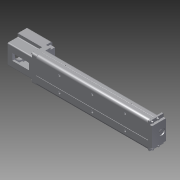
# Autodesk Inventor part: KR45HA-340L-0A0-Body
Saved by Autodesk Inventor 2011 SP1 (Build 150282100, 282)
## iProperties
Created: 2013-10-24
Part Number: KR45HA-340L-0A0-Body
Catalog Web Link: www.cadenas.de
Description: LM Guide Actuator - Body-KR
Vendor: THK
Document SubType Name: Modeling
Designer: PARTuser1
Manufacturer: THK
Density: 1 g/cm^3
Category: PARTsolutions
Company: THK
Title: KR45HA-340L-0A0-Body
Author: Cadenas PARTsolutions
Comments: KR
PSOL_IDENT_0: {$CADENAS_DATA\23d-libs\thk\lm_guide_actuator\type_kr\parts\lm_g_a_kr_body.prj},216 {VTYP=3D},{NB=KR
PSOL_IDENT_1: 45HA-340L-0A0-Body},{LINA=KR45HA-340L-0A0-Body},{NN=LM Guide Actuator - Body},{DATE=10.01.2013 04:45
PSOL_IDENT_2: :24},{GEOMDATE=10.01.2013 04:45:00},{VERSION=},{LINEID=60},{LINESUBID=-1},{WBVAR=LM,TYPE,PC,TOHIF}
PSOL_IDENT_3: {NB=KR45HA-340L-0A0-Body},{LINA=KR45HA-340L-0A0-Body},{KT=DUMMY},{ORDER=KR45H},{XTYPE=6},{LM=340},{L
PSOL_IDENT_4: 1=440},{TYPE=A},{SR=213},{H=70},{G=0},{F=200},{N=3},{N1=2},{LM1=340,440,540,640,740,840,940},{TYPE1=
PSOL_IDENT_5: 'A','B','C','D'},{TYPE2=1},{PC=0},{TOHIF=A0},{TOHIF1='A0','Basic Type (with Housing A, without Inter
PSOL_IDENT_6: mediate flange)','00','Old Basic Type (with Housing A, without Intermediate flange)','0A','Administr
PSOL_IDENT_7: ation number 0A','0B','Administration number 0B','0C','Administration number 0C','0D','Administratio
PSOL_IDENT_8: n number 0D','0F','Administration number 0F'},{TOB=1},{DMTR=64},{A=90},{L=336}
CNS_NT: KR
CNS_NB: KR45HA-340L-0A0-Body
CNS_NBSYN: $ORDER.$TYPE.-$LM.L-$PC.$TOHIF.-Body
CNS_LINA: KR45HA-340L-0A0-Body
CNS_ORDER: KR45H
CNS_XTYPE: 6
CNS_LM: 340
CNS_L1: 440.000
CNS_TYPE: A
CNS_SR: 213.000
CNS_H: 70.000
CNS_G: 0.000
CNS_F: 200.000
CNS_N: 3.000
CNS_N1: 2.000
CNS_LM1: 340,440,540,640,740,840,940
CNS_TYPE1: 'A','B','C','D'
CNS_TYPE2: 1.000
CNS_TOHIF: Basic Type (with Housing A, without Intermediate flange)
CNS_TOHIF1: 'A0','Basic Type (with Housing A, without Intermediate flange)','00','Old Basic Type (with Housing A, without Intermediate flange)','0A','Administration number 0A','0B','Administration number 0B','0C','Administration number 0C','0D','Administration number 0D','0F','Administration number 0F'
CNS_TOB: 1.000
CNS_DMTR: 64.000
CNS_A: 90.000
CNS_L: 336.000
SUPPLIER: THK
ARTICLENO: KR45HA-340L-0A0-Body
BOMINFO: KR45HA-340L-0A0-Body
CREATOR: CADENAS GmbH
Autodesk Inventor part; units mm, degrees
sketch "Sketch_1" plane through (0, 0, 0) normal (1, 0, 0) x (0, 1, 0)
  arc A0 (-22.54, 40) -> (-30.5, 32.04) centre (-22.54, 32.04) ccw
  line L0 (-30.5, 32.04) -> (-30.5, 13)
  line L1 (-30.5, 13) -> (-30, 12.5)
  line L2 (-30, 12.5) -> (-30, -12.5)
  line L3 (-30, -12.5) -> (-30.5, -13)
  line L4 (-30.5, -13) -> (-30.5, -32.04)
  arc A1 (-30.5, -32.04) -> (-22.54, -40) centre (-22.54, -32.04) ccw
  line L5 (-22.54, -40) -> (-15.7, -40)
  line L6 (-15.7, -40) -> (-15.5, -39.8)
  line L7 (-15.5, -39.8) -> (-14.3718, -39.8)
  arc A2 (-12.6282, -39.8) -> (-14.3718, -39.8) centre (-13.5, -41.6) ccw
  line L8 (-12.6282, -39.8) -> (-4.5, -39.8)
  arc A3 (-4.5, -39.8) -> (1.5, -33.8) centre (-4.5, -33.8) ccw
  line L9 (1.5, -33.8) -> (1.5, -29.82)
  line L10 (1.5, -29.82) -> (0.7, -29.02)
  line L11 (0.7, -29.02) -> (-0.6, -29.02)
  line L12 (-0.6, -29.02) -> (-2.75, -31.17)
  line L13 (-2.75, -31.17) -> (-14.25, -31.17)
  line L14 (-14.25, -31.17) -> (-16.4, -29.02)
  line L15 (-16.4, -29.02) -> (-16.5, -29.02)
  arc A4 (-20.5, -25.02) -> (-16.5, -29.02) centre (-16.5, -25.02) ccw
  line L16 (-20.5, -25.02) -> (-20.5, 25.02)
  arc A5 (-16.5, 29.02) -> (-20.5, 25.02) centre (-16.5, 25.02) ccw
  line L17 (-16.5, 29.02) -> (-16.4, 29.02)
  line L18 (-16.4, 29.02) -> (-14.25, 31.17)
  line L19 (-14.25, 31.17) -> (-2.75, 31.17)
  line L20 (-2.75, 31.17) -> (-0.6, 29.02)
  line L21 (-0.6, 29.02) -> (0.7, 29.02)
  line L22 (0.7, 29.02) -> (1.5, 29.82)
  line L23 (1.5, 29.82) -> (1.5, 33.8)
  arc A6 (1.5, 33.8) -> (-4.5, 39.8) centre (-4.5, 33.8) ccw
  line L24 (-4.5, 39.8) -> (-12.6282, 39.8)
  arc A7 (-14.3718, 39.8) -> (-12.6282, 39.8) centre (-13.5, 41.6) ccw
  line L25 (-14.3718, 39.8) -> (-15.5, 39.8)
  line L26 (-15.5, 39.8) -> (-15.7, 40)
  line L27 (-15.7, 40) -> (-22.54, 40)
  constraints: 56 end point, 16 point on circle, 8 centre point
extrude "Extrusion1" add sketch "Sketch_1" along normal blind 340
sketch "Sketch_2" plane through (0, 0, 0) normal (1, 0, 0) x (0, 1, 0)
  line L0 (13, 39.8) -> (-25, 39.8)
  arc A0 (-25, 39.8) -> (-30, 34.8) centre (-25, 34.8) ccw
  line L1 (-30, 34.8) -> (-30, -34.8)
  arc A1 (-30, -34.8) -> (-25, -39.8) centre (-25, -34.8) ccw
  line L2 (-25, -39.8) -> (13, -39.8)
  line L3 (13, -39.8) -> (13, -34)
  line L4 (13, -34) -> (25.75, -34)
  arc A2 (25.75, -34) -> (26.75, -33) centre (25.75, -33) ccw
  line L5 (26.75, -33) -> (26.75, 33)
  arc A3 (26.75, 33) -> (25.75, 34) centre (25.75, 33) ccw
  line L6 (25.75, 34) -> (13, 34)
  line L7 (13, 34) -> (13, 39.8)
  constraints: 16 end point, 8 point on circle, 4 centre point
extrude "Extrusion2" add sketch "Sketch_2" against normal blind 14
sketch "Sketch_3" plane through (0, 0, 0) normal (1, 0, 0) x (0, 1, 0)
  arc A0 (16, 16.52) -> (-16, 16.52) centre (0, -0.0027) ccw
  line L0 (-16, 16.52) -> (-16, -16.52)
  arc A1 (-16, -16.52) -> (16, -16.52) centre (0, 0.0027) ccw
  line L1 (16, -16.52) -> (16, 16.52)
  constraints: 4 end point, 4 point on circle, 2 centre point
extrude "Extrusion3" add sketch "Sketch_3" along normal blind 3.4
sketch "Sketch_4" plane through (0, 0, 0) normal (1, 0, 0) x (0, 1, 0)
  arc A0 (4.5, 22.0454) -> (-16, 15.8193) centre (0, 0) ccw
  line L0 (-16, 15.8193) -> (-16, -15.8193)
  arc A1 (-16, -15.8193) -> (4.5, -22.0454) centre (0, 0) ccw
  line L1 (4.5, -22.0454) -> (4.5, -9.4868)
  arc A2 (4.5, 9.4868) -> (4.5, -9.4868) centre (0, 0) ccw
  line L2 (4.5, 9.4868) -> (4.5, 22.0454)
  constraints: 6 end point, 6 point on circle, 3 centre point
extrude "Extrusion4" add sketch "Sketch_4" along normal blind 12.4
sketch "Sketch_38" plane through (0, 9, 0) normal (0, 1, 0) x (1, 0, 0)
  line L0 (7.4, -15.6) -> (3.4, -15.6)
  line L1 (3.4, -15.6) -> (3.4, -12.1)
  line L2 (3.4, -12.1) -> (7.2, -12.1)
  arc A0 (7.4, -12.3) -> (7.2, -12.1) centre (7.2, -12.3) ccw
  line L3 (7.4, -12.3) -> (7.4, -15.6)
  line L4 (7.4, -15.6) -> (3.4, -15.6)
  constraints: 10 end point, 2 point on circle, 1 centre point
revolve "Revolution1" add sketch "Sketch_38" angle 360 about axis through (7.4, 9, 15.6) along (1, 0, 0)
sketch "Sketch_5" plane through (0, 9, 0) normal (0, 1, 0) x (1, 0, 0)
  line L0 (7.4, 15.6) -> (3.4, 15.6)
  line L1 (3.4, 15.6) -> (3.4, 19.1)
  line L2 (3.4, 19.1) -> (7.2, 19.1)
  arc A0 (7.4, 18.9) -> (7.2, 19.1) centre (7.2, 18.9) ccw
  line L3 (7.4, 18.9) -> (7.4, 15.6)
  line L4 (7.4, 15.6) -> (3.4, 15.6)
  constraints: 10 end point, 2 point on circle, 1 centre point
revolve "Revolution2" add sketch "Sketch_5" angle 360 about axis through (7.4, 9, -15.6) along (1, 0, 0)
sketch "Sketch_7" plane through (340, 0, 0) normal (1, 0, 0) x (0, 0, -1)
  line L0 (-39.8, 11.25) -> (-39.8, -29.25)
  arc A0 (-39.8, -29.25) -> (-39.05, -30) centre (-39.05, -29.25) ccw
  line L1 (-39.05, -30) -> (39.05, -30)
  arc A1 (39.05, -30) -> (39.8, -29.25) centre (39.05, -29.25) ccw
  line L2 (39.8, -29.25) -> (39.8, 11.25)
  arc A2 (39.8, 11.25) -> (39.05, 12) centre (39.05, 11.25) ccw
  line L3 (39.05, 12) -> (-39.05, 12)
  arc A3 (-39.05, 12) -> (-39.8, 11.25) centre (-39.05, 11.25) ccw
  constraints: 8 end point, 8 point on circle, 4 centre point
extrude "Extrusion5" add sketch "Sketch_7" along normal blind 12
sketch "Sketch_23" plane through (0, 0, 0) normal (0, 0, 1) x (1, 0, 0)
  line L0 (343, 0) -> (339, 0)
  line L1 (339, 0) -> (339, 9.5)
  line L2 (339, 9.5) -> (343, 9.5)
  line L3 (343, 9.5) -> (343, 0)
  line L4 (343, 0) -> (339, 0)
  constraints: 10 end point
revolve "Revolution3" cut sketch "Sketch_23" angle 360 about axis through (343, 0, 0) along (1, 0, 0)
sketch "Sketch_8" plane through (340, 0, 0) normal (1, 0, 0) x (0, 0, -1)
  line L0 (-15, -9) -> (15, -9)
  line L1 (15, -9) -> (15, 0)
  line L2 (15, 0) -> (-15, 0)
  line L3 (-15, 0) -> (-15, -9)
  constraints: 8 end point
extrude "Extrusion6" add sketch "Sketch_8" against normal blind 9
sketch "Sketch_9" plane through (0, 0, 0) normal (0, 0, 1) x (1, 0, 0)
  line L0 (344, 0) -> (2, 0)
  line L1 (2, 0) -> (2, 7.5)
  line L2 (2, 7.5) -> (344, 7.5)
  line L3 (344, 7.5) -> (344, 0)
  line L4 (344, 0) -> (2, 0)
  constraints: 10 end point
revolve "Revolution4" add sketch "Sketch_9" angle 360 about axis through (344, 0, 0) along (1, 0, 0)
sketch "Sketch_10" plane through (345, 0, 0) normal (1, 0, 0) x (0, 0, -1)
  line L0 (-45, -35) -> (45, -35)
  line L1 (45, -35) -> (45, 15)
  line L2 (45, 15) -> (31, 15)
  arc A0 (31, 15) -> (30, 14) centre (31, 14) ccw
  line L3 (30, 14) -> (30, -33)
  line L4 (30, -33) -> (-30, -33)
  line L5 (-30, -33) -> (-30, 14)
  arc A1 (-30, 14) -> (-31, 15) centre (-31, 14) ccw
  line L6 (-31, 15) -> (-45, 15)
  line L7 (-45, 15) -> (-45, -35)
  constraints: 16 end point, 4 point on circle, 2 centre point
extrude "Extrusion7" cut sketch "Sketch_10" along normal blind 8
sketch "Sketch_11" plane through (0, -24, 0) normal (0, 1, 0) x (1, 0, 0)
  line L0 (349.8, -35.5) -> (345, -35.5)
  line L1 (345, -35.5) -> (345, -32.365)
  line L2 (345, -32.365) -> (345.5, -32.365)
  line L3 (345.5, -32.365) -> (345.5, -32.475)
  line L4 (345.5, -32.475) -> (346.2, -32.475)
  line L5 (346.2, -32.475) -> (346.2, -32.75)
  line L6 (346.2, -32.75) -> (349.6, -32.75)
  arc A0 (349.8, -32.95) -> (349.6, -32.75) centre (349.6, -32.95) ccw
  line L7 (349.8, -32.95) -> (349.8, -35.5)
  line L8 (349.8, -35.5) -> (345, -35.5)
  constraints: 18 end point, 2 point on circle, 1 centre point
revolve "Revolution5" add sketch "Sketch_11" angle 360 about axis through (349.8, -24, 35.5) along (1, 0, 0)
pattern_linear "Rectangular Pattern1" count 2 spacing 71 along (0, 0, -1) count 2 spacing 17 along (0, 1, 0) of "Revolution5"
sketch "Sketch_39" plane through (0, 0, 0) normal (0, 1, 0) x (-1, 0, 0)
  line L0 (-353, 0) -> (-349, 0)
  line L1 (-350, 0) -> (-350, -4.5)
  line L2 (-350, -4.5) -> (-349.5, -5)
  line L3 (-349.5, -5) -> (-349, -5)
  line L4 (-349, -5) -> (-349, -9.5)
  line L5 (-349, -9.5) -> (-353, -9.5)
  line L6 (-353, -9.5) -> (-353, 0)
  line L7 (-353, 0) -> (-350, 0)
  constraints: 16 end point
revolve "Revolution6" cut sketch "Sketch_39" angle 360 about axis through (353, 0, 0) along (1, 0, 0)
sketch "Sketch_13" plane through (-14, 0, 0) normal (1, 0, 0) x (0, 0, -1)
  line L0 (-39.8, -30) -> (39.8, -30)
  line L1 (39.8, -30) -> (39.8, 27.5)
  arc A0 (39.8, 27.5) -> (34.8, 32.5) centre (34.8, 27.5) ccw
  line L2 (34.8, 32.5) -> (-34.8, 32.5)
  arc A1 (-34.8, 32.5) -> (-39.8, 27.5) centre (-34.8, 27.5) ccw
  line L3 (-39.8, 27.5) -> (-39.8, -30)
  constraints: 8 end point, 4 point on circle, 2 centre point
extrude "Extrusion8" add sketch "Sketch_13" against normal blind 74
sketch "Sketch_14" plane through (-14, 0, 0) normal (1, 0, 0) x (0, 0, -1)
  line L0 (-45, 1) -> (-45, -39)
  line L1 (-45, -39) -> (45, -39)
  line L2 (45, -39) -> (45, 1)
  line L3 (45, 1) -> (32, 1)
  arc A0 (32, 1) -> (30, -1) centre (32, -1) ccw
  line L4 (30, -1) -> (30, -27)
  arc A1 (27, -30) -> (30, -27) centre (27, -27) ccw
  line L5 (27, -30) -> (-27, -30)
  arc A2 (-30, -27) -> (-27, -30) centre (-27, -27) ccw
  line L6 (-30, -27) -> (-30, -1)
  arc A3 (-30, -1) -> (-32, 1) centre (-32, -1) ccw
  line L7 (-32, 1) -> (-45, 1)
  constraints: 16 end point, 8 point on circle, 4 centre point
extrude "Extrusion9" cut sketch "Sketch_14" against normal blind 100
sketch "Sketch_17" plane through (0, 0, 0) normal (0, 1, 0) x (-1, 0, 0)
  arc A0 (74, 8) -> (72, 10) centre (72, 8) ccw
  line L0 (72, 10) -> (25, 10)
  arc A1 (25, 10) -> (23, 8) centre (25, 8) ccw
  line L1 (23, 8) -> (23, -8)
  arc A2 (23, -8) -> (25, -10) centre (25, -8) ccw
  line L2 (25, -10) -> (72, -10)
  arc A3 (72, -10) -> (74, -8) centre (72, -8) ccw
  line L3 (74, -8) -> (74, 8)
  constraints: 8 end point, 8 point on circle, 4 centre point
extrude "Extrusion10" cut sketch "Sketch_17" against normal blind 35
sketch "Sketch_15" plane through (0, -24.2, 0) normal (0, 1, 0) x (1, 0, 0)
  arc A0 (-74, -24.9) -> (-72.9, -26) centre (-72.9, -24.9) ccw
  line L0 (-72.9, -26) -> (-24.1, -26)
  arc A1 (-24.1, -26) -> (-23, -24.9) centre (-24.1, -24.9) ccw
  line L1 (-23, -24.9) -> (-23, 24.9)
  arc A2 (-23, 24.9) -> (-24.1, 26) centre (-24.1, 24.9) ccw
  line L2 (-24.1, 26) -> (-72.9, 26)
  arc A3 (-72.9, 26) -> (-74, 24.9) centre (-72.9, 24.9) ccw
  line L3 (-74, 24.9) -> (-74, -24.9)
  constraints: 8 end point, 8 point on circle, 4 centre point
extrude "Extrusion11" cut sketch "Sketch_15" along normal blind 60
sketch "Sketch_24" plane through (0, 0, 0) normal (0, 1, 0) x (-1, 0, 0)
  arc A0 (74, 28.9) -> (72.9, 30) centre (72.9, 28.9) ccw
  line L0 (72.9, 30) -> (24.1, 30)
  arc A1 (24.1, 30) -> (23, 28.9) centre (24.1, 28.9) ccw
  line L1 (23, 28.9) -> (23, -28.9)
  arc A2 (23, -28.9) -> (24.1, -30) centre (24.1, -28.9) ccw
  line L2 (24.1, -30) -> (72.9, -30)
  arc A3 (72.9, -30) -> (74, -28.9) centre (72.9, -28.9) ccw
  line L3 (74, -28.9) -> (74, 28.9)
  constraints: 8 end point, 8 point on circle, 4 centre point
extrude "Extrusion12" cut sketch "Sketch_24" along normal blind 40
sketch "Sketch_18" plane through (0, 0, 0) normal (0, 0, 1) x (1, 0, 0)
  line L0 (-74, 0) -> (-89, 0)
  line L1 (-89, 0) -> (-89, 25)
  line L2 (-89, 25) -> (-84.5, 25)
  line L3 (-84.5, 25) -> (-84.5, 22)
  line L4 (-84.5, 22) -> (-74, 22)
  line L5 (-74, 22) -> (-74, 0)
  line L6 (-74, 0) -> (-89, 0)
  constraints: 14 end point
revolve "Revolution7" cut sketch "Sketch_18" angle 360 about axis through (-74, 0, 0) along (1, 0, 0)
sketch "Sketch_19" plane through (0, -24, 0) normal (0, 1, 0) x (1, 0, 0)
  line L0 (-14, -35.5) -> (-18, -35.5)
  line L1 (-18, -35.5) -> (-18, -32.2)
  arc A0 (-17.8, -32) -> (-18, -32.2) centre (-17.8, -32.2) ccw
  line L2 (-17.8, -32) -> (-14, -32)
  line L3 (-14, -32) -> (-14, -35.5)
  line L4 (-14, -35.5) -> (-18, -35.5)
  constraints: 10 end point, 2 point on circle, 1 centre point
revolve "Revolution8" add sketch "Sketch_19" angle 360 about axis through (-14, -24, 35.5) along (1, 0, 0)
pattern_linear "Rectangular Pattern2" count 2 spacing 71 along (0, 0, -1) count 2 spacing 17 along (0, 1, 0) of "Revolution8"
sketch "Sketch_21" plane through (0, 0, 0) normal (0, 0, 1) x (1, 0, 0)
  line L0 (-23, 0) -> (-51, 0)
  line L1 (-51, 0) -> (-51, 4)
  line L2 (-51, 4) -> (-50, 5)
  line L3 (-50, 5) -> (-33, 5)
  line L4 (-33, 5) -> (-32, 6)
  line L5 (-32, 6) -> (-31, 6)
  line L6 (-31, 6) -> (-31, 10)
  line L7 (-31, 10) -> (-30, 11)
  line L8 (-30, 11) -> (-24.5, 11)
  line L9 (-24.5, 11) -> (-23.5, 10)
  line L10 (-23.5, 10) -> (-23.5, 8.8)
  line L11 (-23.5, 8.8) -> (-23, 8.8)
  line L12 (-23, 8.8) -> (-23, 0)
  line L13 (-23, 0) -> (-51, 0)
  constraints: 28 end point
revolve "Revolution9" add sketch "Sketch_21" angle 360 about axis through (-23, 0, 0) along (1, 0, 0)
sketch "Sketch_22" plane through (-23, 0, 0) normal (1, 0, 0) x (0, 0, -1)
  circle A0 centre (0, 0) radius 14
  line L0 (-12.7279, 0) -> (0, -12.7279)
  line L1 (0, -12.7279) -> (12.7279, 0)
  line L2 (12.7279, 0) -> (0, 12.7279)
  line L3 (0, 12.7279) -> (-12.7279, 0)
  constraints: 8 end point, 1 centre point
extrude "Extrusion13" cut sketch "Sketch_22" against normal blind 15
sketch "Sketch_37" plane through (0, 0, 0) normal (0, 0, 1) x (1, 0, 0)
  line L0 (-27.25, 10) -> (-27.25, 11.5)
  line L1 (-27.25, 11.5) -> (-24.5, 11.5)
  line L2 (-24.5, 11.5) -> (-24.5, 10)
  line L3 (-24.5, 10) -> (-27.25, 10)
  line L4 (-27.25, 10) -> (-27.25, 11.5)
  constraints: 10 end point
revolve "Revolution10" cut sketch "Sketch_37" angle 360 about axis through (-27.25, 10, 0) along (0, -1, 0)
sketch "Sketch24" plane through (340, -15.5, -39.8) normal (0, 0, -1) x (-1, 0, 0)
  point P0 (270, 4)
hole "Drilling 4" at (70, -11.5, -39.8) direction (0, 0, 1) diameter 2.1129 depth 5 tip angle 140 countersink diameter 2.6 countersink angle 90 thread size "M2.6x0.45" class "6H" standard "ISO Metric profile"
pattern_linear "Rectangular Pattern3" count 2 spacing 200 along (1, 0, 0) of "Drilling 4"
sketch "Sketch25" plane through (0, -15.5, 39.8) normal (0, 0, 1) x (1, 0, 0)
  point P0 (70, 4)
hole "Drilling 5" at (70, -11.5, 39.8) direction (0, 0, -1) diameter 2.1129 depth 5 tip angle 140 countersink diameter 2.6 countersink angle 90 thread size "M2.6x0.45" class "6H" standard "ISO Metric profile"
pattern_linear "Rectangular Pattern4" count 2 spacing 200 along (1, 0, 0) of "Drilling 5"
sketch "Sketch_29" plane through (70, 0, 0) normal (1, 0, 0) x (0, 0, -1)
  line L0 (-23, -18) -> (-23, -31)
  line L1 (-23, -31) -> (-26.3, -31)
  line L2 (-26.3, -31) -> (-26.3, -27)
  line L3 (-26.3, -27) -> (-28.5, -27)
  line L4 (-28.5, -27) -> (-28.5, -18)
  line L5 (-28.5, -18) -> (-23, -18)
  line L6 (-23, -18) -> (-23, -31)
  constraints: 14 end point
revolve "Revolution11" cut sketch "Sketch_29" angle 360 about axis through (70, -18, 23) along (0, 1, 0)
pattern_linear "Rectangular Pattern5" count 3 spacing 100 along (1, 0, 0) of "Revolution11"
sketch "Sketch_31" plane through (70, 0, 0) normal (1, 0, 0) x (0, 0, -1)
  line L0 (23, -18) -> (23, -31)
  line L1 (23, -31) -> (19.7, -31)
  line L2 (19.7, -31) -> (19.7, -27)
  line L3 (19.7, -27) -> (17.5, -27)
  line L4 (17.5, -27) -> (17.5, -18)
  line L5 (17.5, -18) -> (23, -18)
  line L6 (23, -18) -> (23, -31)
  constraints: 14 end point
revolve "Revolution12" cut sketch "Sketch_31" angle 360 about axis through (70, -18, -23) along (0, 1, 0)
pattern_linear "Rectangular Pattern6" count 3 spacing 100 along (1, 0, 0) of "Revolution12"
sketch "Sketch_46" plane through (12.4, 0, 0) normal (1, 0, 0) x (0, 0, -1)
  line L0 (15.8, 5) -> (15.8, -0.5)
  arc A0 (15.8, -0.5) -> (16.3, -1) centre (16.3, -0.5) ccw
  line L1 (16.3, -1) -> (23.8, -1)
  line L2 (23.8, -1) -> (23.8, 5)
  line L3 (23.8, 5) -> (15.8, 5)
  constraints: 8 end point, 2 point on circle, 1 centre point
extrude "Extrusion14" cut sketch "Sketch_46" against normal blind 8
sketch "Sketch29" plane through (-88, 0, 0) normal (-1, 0, 0) x (0, 0, 1)
  point P0 (24.7487, -24.7487)
hole "Drilling 8" at (-88, -24.7487, 24.7487) direction (1, 0, 0) diameter 4.134 depth 12 tip angle 120 countersink diameter 5 countersink angle 90 thread size "M5x0.8" class "6H" standard "ISO Metric profile"
pattern_linear "Rectangular Pattern7" count 2 spacing 49.4975 along (0, 0, -1) count 2 spacing 49.4975 along (0, 1, 0) of "Drilling 8"
ref_plane "body_dummy_XY" through (0, 0, 0) normal (1, 0, 0) x (0, 0, -1)
ref_plane "body_dummy_YZ" through (0, 0, 0) normal (0, 0, -1) x (0, 1, 0)
ref_plane "body_dummy_ZX" through (0, 0, 0) normal (0, 1, 0) x (1, 0, 0)
ref_plane "body_flange_XY" through (-88, 0, 0) normal (1, 0, 0) x (0, 0, -1)
ref_plane "body_flange_YZ" through (-88, 0, 0) normal (0, 0, -1) x (0, 1, 0)
ref_plane "body_flange_ZX" through (-88, 0, 0) normal (0, 1, 0) x (1, 0, 0)
ref_plane "body_pc_XY" through (-7, 26.75, 0) normal (1, 0, 0) x (0, 0, -1)
ref_plane "body_pc_YZ" through (-7, 26.75, 0) normal (0, 0, -1) x (0, 1, 0)
ref_plane "body_pc_ZX" through (-7, 26.75, 0) normal (0, 1, 0) x (1, 0, 0)
ref_plane "body_sensor_rail_XY" through (170, -11.5, 39.8) normal (0, 0, 1) x (1, 0, 0)
ref_plane "body_sensor_rail_YZ" through (170, -11.5, 39.8) normal (1, 0, 0) x (0, 1, 0)
ref_plane "body_sensor_rail_ZX" through (170, -11.5, 39.8) normal (0, 1, 0) x (0, 0, 1)
ref_plane "body_sensor_rail2_XY" through (170, -11.5, -39.8) normal (0, 0, 1) x (1, 0, 0)
ref_plane "body_sensor_rail2_YZ" through (170, -11.5, -39.8) normal (1, 0, 0) x (0, 1, 0)
ref_plane "body_sensor_rail2_ZX" through (170, -11.5, -39.8) normal (0, 1, 0) x (0, 0, 1)
ref_plane "body_slider_XY" through (12.4, 0, 0) normal (1, 0, 0) x (0, 0, -1)
ref_plane "body_slider_YZ" through (12.4, 0, 0) normal (0, 0, -1) x (0, 1, 0)
ref_plane "body_slider_ZX" through (12.4, 0, 0) normal (0, 1, 0) x (1, 0, 0)
ref_plane "body_slider2_XY" through (331, 0, 0) normal (1, 0, 0) x (0, 0, -1)
ref_plane "body_slider2_YZ" through (331, 0, 0) normal (0, 0, -1) x (0, 1, 0)
ref_plane "body_slider2_ZX" through (331, 0, 0) normal (0, 1, 0) x (1, 0, 0)
body "Solid1"
